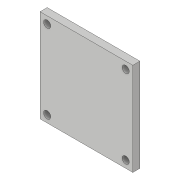
# Autodesk Inventor part: M
Saved by Autodesk Inventor 2019 (Build 230136000, 136)
## iProperties
Created: 2019-10-08
Part Number: M
Material: Generic
Document SubType Name: Modeling
Designer: Admin
Density: 1 g/cm^3
Appearance: Default
Author: Admin
Autodesk Inventor part; units mm, degrees
ref_plane "YZ Plane" through (0, 0, 0) normal (1, 0, 0) x (0, 1, 0)
ref_plane "XZ Plane" through (0, 0, 0) normal (0, 1, 0) x (-1, 0, 0)
ref_plane "XY Plane" through (0, 0, 0) normal (0, 0, 1) x (1, 0, 0)
sketch "Sketch1" plane through (0, 0, 0) normal (0, 0, 1) x (1, 0, 0)
  line L0 (0, 0) -> (130, 0)
  line L1 (130, 0) -> (130, 130)
  line L2 (130, 130) -> (0, 130)
  line L3 (0, 130) -> (0, 0)
  line L4 (0, 130) -> (19.05, 130)
  line L5 (0, 130) -> (3.175, 130)
  dimension "d0" = 130
  dimension "d1" = 130
  constraints: 12 end point, 2 parallel, 2 point on line, 1 horizontal, 1 perpendicular
  measures "d0" distance of L2.end L1.end
  measures "d1" distance of L1.end L0.end
extrude "Extrusion1" add sketch "Sketch1" along normal blind 10
sketch "Sketch2" plane through (0, 0, 10) normal (0, 0, 1) x (1, 0, 0)
  line L0 (130, 130) -> (0, 130) projected
  line L1 (0, 130) -> (10, 130)
  line L2 (10, 130) -> (10, 10)
  line L3 (10, 10) -> (120, 10)
  line L4 (120, 10) -> (120, 120)
  line L5 (120, 120) -> (10, 120)
  circle A0 centre (10, 120) radius 5
  circle A1 centre (120, 120) radius 5
  circle A2 centre (120, 10) radius 5
  circle A3 centre (10, 10) radius 5
  point P0 (0, 0)
  dimension "d4" = 10
  dimension "d5" = 120
  dimension "d6" = 110
  dimension "d7" = 110
  dimension "d8" = 110
  dimension "d9" = 10
  dimension "d10" = 10
  dimension "d11" = 10
  dimension "d12" = 10
  constraints: 10 end point, 4 centre point, 4 coincident, 3 perpendicular, 2 point on line
  measures "d4" distance of L0.end L1.end
  measures "d5" distance of L1.end L2.end
  measures "d6" distance of L2.end L3.end
  measures "d7" distance of L3.end L4.end
  measures "d8" distance of L4.end L5.end
  measures "d9" diameter of A0
  measures "d10" diameter of A1
  measures "d11" diameter of A2
  measures "d12" diameter of A3
extrude "Extrusion2" cut sketch "Sketch2" against normal through all contours A0 L5 L2 | L2 A0 | L5 A0 L2 | A1 L4 L5 | L5 L4 A1 | A3 L3 L2 | L2 L3 A3 | A2 L3 L4 | L4 L3 A2
sketch "Sketch3" plane through (0, 0, 10) normal (0, 0, 1) x (1, 0, 0)
  line L0 (0, 0) -> (65, 0)
  line L1 (0, 0) -> (130, 0) projected
  line L2 (65, 0) -> (65, 30)
  circle A0 centre (65, 30) radius 5.5
  line L3 (130, 130) -> (0, 130) projected
  line L4 (0, 130) -> (65, 130)
  line L5 (65, 130) -> (65, 95)
  circle A1 centre (65, 95) radius 25
  circle A2 centre (65, 95) radius 30
  circle A3 centre (49.2125, 109.5375) radius 8.0947
  circle A4 centre (50.8, 84.1375) radius 8.5489
  circle A5 centre (76.2, 79.375) radius 8.5489
  circle A6 centre (82.55, 101.4428) radius 8.1613
  circle A7 centre (69.85, 112.5) radius 7.6806
  circle A8 centre (84.7489, 96.8375) radius 7.4376
  dimension "d15" = 65
  dimension "d16" = 30
  dimension "d17" = 11
  dimension "d18" = 65
  dimension "d19" = 35
  dimension "d23" = 50
  dimension "d24" = 60
  constraints: 9 centre point, 8 end point, 3 coincident, 2 midpoint, 2 perpendicular
  measures "d15" distance of L0.start L0.end
  measures "d16" distance of L0.end L2.end
  measures "d17" diameter of A0
  measures "d18" distance of L3.end L4.end
  measures "d19" distance of L4.end L5.end
  measures "d23" diameter of A1
  measures "d24" diameter of A2
extrude "Extrusion3" [suppressed]
body "Solid1"
